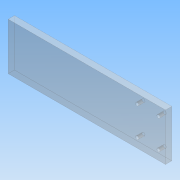
# Autodesk Inventor part: Base
Saved by Autodesk Inventor 2016 (Build 200138000, 138)
## iProperties
Created: 2015-08-01
Part Number: Base
Material: Generic
Document SubType Name: Modeling
Designer: Openlab
Density: 1 g/cm^3
Appearance: Polycarbonate - Clear
Author: Openlab
Autodesk Inventor part; units mm, degrees
ref_plane "YZ Plane" through (0, 0, 0) normal (1, 0, 0) x (0, 1, 0)
ref_plane "XZ Plane" through (0, 0, 0) normal (0, 1, 0) x (-1, 0, 0)
ref_plane "XY Plane" through (0, 0, 0) normal (0, 0, 1) x (1, 0, 0)
sketch "Sketch1" plane through (0, 0, 0) normal (0, 1, 0) x (-1, 0, 0)
  line L0 (0, 0) -> (200, 0)
  line L1 (200, 0) -> (200, -60)
  line L2 (200, -60) -> (0, -60)
  line L3 (0, -60) -> (0, 0)
  dimension "d0" = 200
  dimension "d1" = 60
  constraints: 8 end point, 2 parallel, 1 horizontal, 1 perpendicular
  measures "d0" distance of L1.end L2.end
  measures "d1" distance of L0.end L1.end
extrude "Extrusion1" add sketch "Sketch1" along normal blind 8
sketch "Sketch2" plane through (0, 8, 0) normal (0, 1, 0) x (1, 0, 0)
  line L0 (-40, 7.5) -> (-40, 52.5)
  line L1 (-35, 42.75) -> (-35, 34.25)
  line L2 (-35, 34.25) -> (-34, 34.25)
  line L3 (-34, 34.25) -> (-34, 42.75)
  line L4 (-34, 42.75) -> (-35, 42.75)
  line L5 (-34, 25.75) -> (-35, 25.75)
  line L6 (-35, 25.75) -> (-35, 17.25)
  line L7 (-35, 17.25) -> (-34, 17.25)
  line L8 (-34, 17.25) -> (-34, 25.75)
  line L9 (-40, 7.5) -> (-5, 7.5)
  line L10 (-5, 52.5) -> (-40, 52.5)
  line L11 (-23.5275, 30) -> (-17.7049, 30) construction
  line L12 (-5, 52.5) -> (-5, 7.5)
  circle A0 centre (-36, 11.5) radius 1.5
  circle A1 centre (-9, 11.5) radius 1.5
  circle A2 centre (-36, 48.5) radius 1.5
  circle A3 centre (-9, 48.5) radius 1.5
  line L13 (-200, 0) -> (0, 0) construction
  line L14 (0, 0) -> (0, 60) construction
  point P0 (-35.5, 13)
  point P1 (-35.5, 30)
  point P2 (-35.5, 47)
  dimension "d4" = 8.5
  dimension "d5" = 1
  dimension "d6" = 5
  dimension "d7" = 17
  dimension "d8" = 17
  dimension "d9" = 4.25
  dimension "d10" = 4.25
  dimension "d11" = 4.5
  dimension "d12" = 35
  dimension "d13" = 45
  dimension "d14" = 3
  dimension "d15" = 4
  dimension "d16" = 4
  dimension "d17" = 4
  dimension "d18" = 4
  dimension "d19" = 7.5
  dimension "d20" = 5
  constraints: 26 end point, 7 perpendicular, 4 centre point, 4 coincident, 4 vertical alignment, 3 equal radius, 2 equal length, 2 horizontal alignment, 2 parallel, 2 point on line, 1 collinear, 1 other
  measures "d4" distance of L7.end L5.start
  measures "d5" distance of L6.end L7.end
  measures "d6" distance between parallel lines of L0 L6
  measures "d7" distance of point (-35.5, 30) point (-35.5, 13)
  measures "d8" distance of point (-35.5, 47) point (-35.5, 30)
  measures "d9" distance from line of L7 point (-35.5, 13)
  measures "d10" distance from line of point (-35.5, 30) L2
  measures "d11" distance from line of L0 point (-35.5, 47)
  measures "d12" distance of L0.start L9.end
  measures "d13" distance of L0.start L0.end
  measures "d14" diameter of A0
  measures "d15" distance from line of L0 A0.centre
  measures "d16" distance from line of L9 A0.centre
  measures "d17" distance from line of L10 A3.centre
  measures "d18" distance from line of L12 A3.centre
  measures "d19" distance between parallel lines of L13 L9
  measures "d20" distance between parallel lines of L14 L12
hole "Hole1" at (-36, 8, -11.5) at (-36, 8, -48.5) at (-9, 8, -11.5) at (-9, 8, -48.5) direction (0, -1, 0) diameter 4 end through all
body "Solid1"
